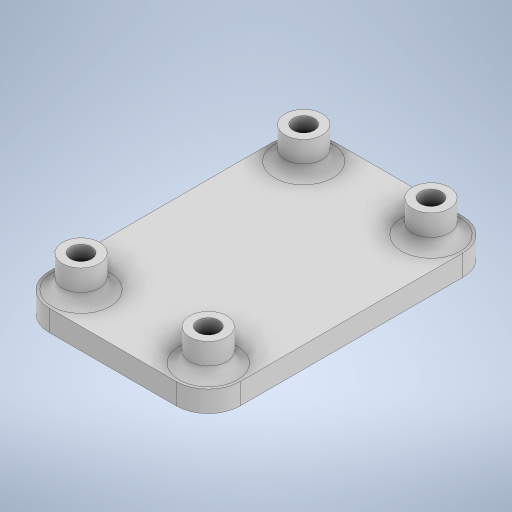
# Autodesk Inventor part: drzak_kamery
Saved by Autodesk Inventor 2024 (Build 280153000, 153)
## iProperties
Created: 2024-05-02
Part Number: drzak_kamery
Material: Všeobecné
Document SubType Name: Modeling
Designer: eliasla
Density: 1 g/cm^3
Appearance: Výchozí
Author: eliasla
Autodesk Inventor part; units mm, degrees
ref_plane "YZ Plane" through (0, 0, 0) normal (1, 0, 0) x (0, 1, 0)
ref_plane "XZ Plane" through (0, 0, 0) normal (0, 1, 0) x (-1, 0, 0)
ref_plane "XY Plane" through (0, 0, 0) normal (0, 0, 1) x (1, 0, 0)
sketch "Náčrt1" plane through (0, 0, 0) normal (0, 0, 1) x (1, 0, 0)
  circle A0 centre (0, 0) radius 1
  circle A1 centre (12, 0) radius 1
  circle A2 centre (0, 21) radius 1
  circle A3 centre (12, 21) radius 1
  line L0 (12, 24) -> (0, 24)
  arc A4 (0, 24) -> (-3, 21) centre (0, 21) ccw
  line L1 (-3, 21) -> (-3, 0)
  arc A5 (-3, 0) -> (0, -3) centre (0, 0) ccw
  line L2 (0, -3) -> (12, -3)
  arc A6 (12, -3) -> (15, 0) centre (12, 0) ccw
  line L3 (15, 0) -> (15, 21)
  arc A7 (15, 21) -> (12, 24) centre (12, 21) ccw
  dimension "d0" = 2
  dimension "d1" = 10
  constraints: 8 centre point, 8 end point, 8 point on circle, 1 coincident
  measures "d0" diameter of A0
extrude "Vysunutí1" add sketch "Náčrt1" along normal blind 2
sketch "Náčrt2" plane through (0, 0, 2) normal (0, 0, 1) x (1, 0, 0)
  circle A0 centre (0, 0) radius 1 projected
  circle A1 centre (0, 0) radius 1
  line L0 (0, -3) -> (12, -3) projected
  circle A2 centre (12, 0) radius 1
  line L1 (-3, 21) -> (-3, 0) projected
  line L2 (15, 0) -> (15, 21) projected
  circle A3 centre (0, 21) radius 1
  circle A4 centre (12, 21) radius 1
  circle A5 centre (0, 21) radius 1.75
  circle A6 centre (12, 21) radius 1.75
  circle A7 centre (12, 0) radius 1.75
  circle A8 centre (0, 0) radius 1.75
  dimension "d10" = 0.75
  dimension "d11" = 0.75
  dimension "d12" = 0.75
  dimension "d14" = 0.75
  constraints: 8 centre point, 1 coincident
  measures "d10" radial gap between concentric circles of A3 A5
  measures "d11" radial gap between concentric circles of A4 A6
  measures "d12" radial gap between concentric circles of A2 A7
  measures "d14" radial gap between concentric circles of A0 A8
extrude "Vysunutí2" add sketch "Náčrt2" along normal blind 3
fillet "Zaoblení1" radius 1 1 edges at (-1.75, 0, 2)
fillet "Zaoblení2" radius 1 3 edges at (-1.75, 21, 2) (10.25, 21, 2) (10.25, 0, 2)
